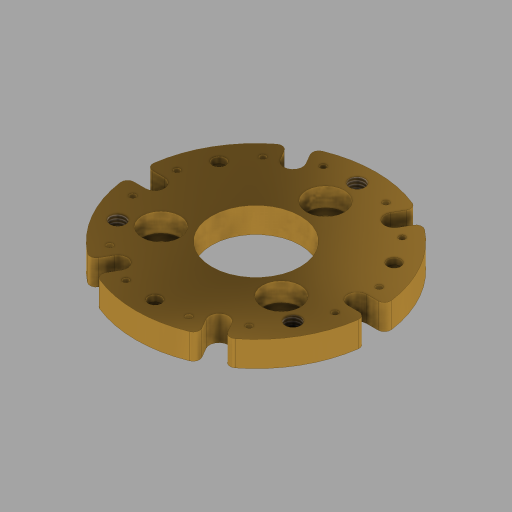
# Autodesk Inventor part: Insert_flange_Top
Saved by Autodesk Inventor 2024 (Build 280153020, 153B)
## iProperties
Created: 2023-09-24
Part Number: Insert_flange_Top
Material: Brass
Document SubType Name: Modeling
Designer: schanen
Density: 8.49 g/cm^3
Appearance: Brass - Polished
CD: 16.000 mm
OD: 4.000 mm
WA: 0.300 mm
THR: 3.000 mm
Author: schanen
Autodesk Inventor part; units mm, degrees
ref_plane "YZ Plane" through (0, 0, 0) normal (1, 0, 0) x (0, 1, 0)
ref_plane "XZ Plane" through (0, 0, 0) normal (0, 1, 0) x (-1, 0, 0)
ref_plane "XY Plane" through (0, 0, 0) normal (0, 0, 1) x (1, 0, 0)
sketch "Sketch1" plane through (0, 0, 0) normal (0, 0, 1) x (1, 0, 0)
  line L0 (-7, 0) -> (-19, 0)
  line L1 (-19, 0) -> (-19, 4)
  line L2 (-19, 4) -> (-7, 4)
  line L3 (-7, 4) -> (-7, 0)
  line L4 (0, -0.8) -> (0, 4.8) projected
  point P0 (0, 0)
  dimension "d2" = 4
  dimension "d60" = 7
  dimension "d61" = 19
  constraints: 8 end point, 2 parallel, 1 horizontal, 1 horizontal alignment, 1 perpendicular
  measures "d2" distance of L0.end L1.end
  measures "d60" distance between parallel lines of L4 L3
  measures "d61" distance between parallel lines of L4 L1
revolve "Revolution1" add sketch "Sketch1" angle 360 about axis through (0, -10, 0) along (0, 1, 0)
sketch "Sketch3" plane through (0, 4, 0) normal (0, 1, 0) x (1, 0, 0)
  point P0 (0, 0)
  point P1 (0, 11)
  dimension "d16" = 11
  measures "d16" distance of point (0, 0) point (0, 11)
hole "Hole2" at (0, 4, -11) direction (0, -1, 0) diameter 3 end through all counterbore diameter 6 counterbore depth 3
pattern_circular "Circular Pattern1" count 3 over 360 about axis through (0, 2, 0) along (0, 1, 0) of "Hole2"
sketch "Sketch4" plane through (0, 0, 0) normal (0, -1, 0) x (1, 0, 0)
  point P0 (0, 0)
  point P1 (0, 16)
  dimension "d27" = 16
  measures "d27" distance of point (0, 0) point (0, 16)
hole "Hole3" at (0, 0, 16) direction (0, 1, 0) diameter 2.1 end through all counterbore diameter 4.2 counterbore depth 3
pattern_circular "Circular Pattern2" count 3 over 360 about axis through (0, 2, 0) along (0, 1, 0) of "Hole3"
sketch "Sketch5" plane through (0, 0, 0) normal (0, -1, 0) x (1, 0, 0)
  circle A0 centre (-13.8564, -8) radius 1.05 projected
  circle A1 centre (0, 0) radius 16 construction
  circle A2 centre (-16, 0) radius 1.5
  line L0 (-16, 1.5) -> (-18.9407, 1.5)
  circle A3 centre (0, 0) radius 19 projected
  line L1 (-16, -1.5) -> (-18.9407, -1.5)
  arc A4 (-18.9407, 1.5) -> (-18.9407, -1.5) centre (0, 0) ccw
  circle A5 centre (-16, 3.5) radius 0.5
  circle A6 centre (-16, -3.5) radius 0.5
  dimension "d38" = 3
  dimension "d42" = 1
  dimension "d43" = 2
  dimension "d44" = 1
  dimension "d45" = 2
  constraints: 8 point on circle, 5 centre point, 4 end point, 2 coincident, 1 horizontal, 1 horizontal alignment, 1 parallel, 1 tangent
  measures "d38" diameter of A2
  measures "d42" diameter of A5
  measures "d43" distance of A5.centre L0.start
  measures "d44" diameter of A6
  measures "d45" distance of L1.start A6.centre
extrude "Extrusion1" cut sketch "Sketch5" against normal through all contours A2 | A2 L1 A3 L0 | A5 | A6 picked at (-18.4455, -0.8441)
fillet "Fillet1" radius 1 2 edges at (-18.9407, 2, -1.5) (-18.9407, 2, 1.5)
pattern_circular "Circular Pattern3" count 2 over 60 about axis through (0, 2, 0) along (0, 1, 0) of "Fillet1", "Extrusion1"
sketch "Sketch7" plane through (-16, 0, 0) normal (0, -1, 0) x (1, 0, 0)
  arc A0 (0, -1.5) -> (0, 1.5) centre (0, 0) ccw projected
  circle A1 centre (16, 0) radius 16 construction
  point P0 (16, 0)
  point P1 (2.1436, 8)
  dimension "d49" = 30
  constraints: 2 point on circle, 1 centre point, 1 coincident
hole "Hole4" at (-13.8564, 0, 8) direction (0, 1, 0) diameter 2.459 end through all thread size "M3x0.5" class "6H" standard "ISO Metric profile"
pattern_circular "Circular Pattern4" count 3 over 360 about axis through (0, 2, 0) along (0, 1, 0) of "Extrusion1", "Fillet1", "Circular Pattern3", "Hole4"
equation "\"d27\" = CD"
equation "\"d45\" = d43"
equation "\"CD\" = 16"
equation "\"OD\" = 4"
equation "\"WA\" = 0.3"
equation "\"THR\" = 3"
body "Solid1"
